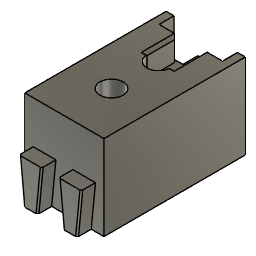
Connector_piece (Autodesk Fusion 360 design; units mm, degrees)
Autodesk Fusion 360 part; units mm, degrees
note: some values were not read from the file. Set by a fixed rule: which sketch regions a step uses.
sketch "Sketch1" plane through (0, 0, 0) normal (0, 1, 0) x (1, 0, 0)
  line L0 (0, 0) -> (28, 0)
  line L1 (28, 0) -> (28, -30)
  line L2 (28, -30) -> (0, -30)
  line L3 (0, -30) -> (0, 0)
  dimension "d1" = 28
  dimension "d2" = 30
  constraint horizontal L0
  constraint vertical L1
  constraint horizontal L2
  constraint vertical L3
  constraint coincident L0.start L3.end
  measures "d1" distance of L0.start L0.end
  measures "d2" distance of L0.start L2.end
extrude "Extrude1" add sketch "Sketch1" along normal blind 50
sketch "Sketch3" plane through (0, 0, 30) normal (0, 0, 1) x (-1, 0, 0)
  line L0 (0, 0) -> (-28, 0)
  line L1 (-28, 0) -> (-28, -50)
  line L2 (-28, -50) -> (0, -50)
  line L3 (0, -50) -> (0, 0)
  line L4 (0, -16.6667) -> (-28, -16.6667)
  line L5 (0, -33.3333) -> (-28, -33.3333)
  circle A0 centre (-14, -33.3333) radius 2
  circle A1 centre (-14, -16.6667) radius 2
  circle A2 centre (-14, -16.6667) radius 4.1
  circle A3 centre (-14, -33.3333) radius 4.1
  dimension "d25" = 16.6667
  dimension "d26" = 16.6667
  dimension "d27" = 4
  dimension "d28" = 4
  dimension "d29" = 8.2
  dimension "d30" = 8.2
  constraint coincident L3 L4.start
  constraint coincident L1 L4.end
  constraint perpendicular L1 L4
  constraint coincident L3 L5.start
  constraint coincident L1 L5.end
  constraint perpendicular L1 L5
  constraint midpoint L5 A0.centre
  constraint midpoint L4 A1.centre
  constraint concentric A1 A2
  constraint concentric A0 A3
  measures "d25" distance of L0 L4
  measures "d26" distance of L2 L5
  measures "d27" diameter of A0
  measures "d28" diameter of A1
  measures "d29" diameter of A2
  measures "d30" diameter of A3
extrude "Extrude5" cut sketch "Sketch3" against normal blind 30 contours L4 A1 | L4 A1 | L5 A0 | L5 A0
sketch "Sketch2" plane through (0, 50, 0) normal (0, 1, 0) x (-1, 0, 0)
  line L0 (0, 30) -> (-28, 30)
  line L1 (-28, 30) -> (-28, 0)
  line L2 (-28, 0) -> (0, 0)
  line L3 (0, 0) -> (0, 30)
  line L4 (-28, 30) -> (-14, 30) construction
  line L5 (-14, 30) -> (-14, 0) construction
  line L6 (-14, 0) -> (-28, 0) construction
  line L7 (-28, 0) -> (-28, 30) construction
  line L8 (-21, 30) -> (-21, 0) construction
  line L9 (-21, 0) -> (-23.5, 0)
  line L10 (-21, 0) -> (-18.5, 0)
  line L11 (-21, 15) -> (-25, 15)
  line L12 (-25, 15) -> (-23.5, 0)
  line L13 (-21, 0) -> (-18.5, 0)
  line L14 (-21, 0) -> (-23.5, 0)
  line L15 (-17, 15) -> (-18.5, 0)
  line L16 (-21, 15) -> (-17, 15)
  line L17 (-11, 15) -> (-9.5, 0)
  line L18 (-7, 15) -> (-11, 15)
  line L19 (-7, 15) -> (-3, 15)
  line L20 (-3, 15) -> (-4.5, 0)
  line L21 (-7, 0) -> (-4.5, 0)
  line L22 (-7, 0) -> (-9.5, 0)
  line L23 (-21, 15.5) -> (-16.4475, 15.5)
  line L24 (-16.4475, 15.5) -> (-18.0475, -0.5)
  line L25 (-21, -0.5) -> (-18.0475, -0.5)
  line L26 (-21, -0.5) -> (-23.9525, -0.5)
  line L27 (-25.5525, 15.5) -> (-23.9525, -0.5)
  line L28 (-21, 15.5) -> (-25.5525, 15.5)
  line L29 (-7, -0.5) -> (-9.9525, -0.5)
  line L30 (-11.5525, 15.5) -> (-9.9525, -0.5)
  line L31 (-7, 15.5) -> (-11.5525, 15.5)
  line L32 (-7, 15.5) -> (-2.4475, 15.5)
  line L33 (-2.4475, 15.5) -> (-4.0475, -0.5)
  line L34 (-7, -0.5) -> (-4.0475, -0.5)
  line L35 (-25.5525, 15.5) -> (-25.5525, 30)
  line L36 (-2.4475, 15.5) -> (-2.4475, 30)
  line L37 (-16.4475, 15.5) -> (-16.4475, 30)
  line L38 (-11.5525, 15.5) -> (-11.5525, 30)
  line L39 (-28, 30) -> (-28, 22)
  line L40 (0, 30) -> (0, 22)
  line L41 (0, 22) -> (-9.2, 22)
  line L42 (-28, 22) -> (-18.8, 22)
  line L43 (-18.8, 22) -> (-18.8, 30)
  line L44 (-9.2, 22) -> (-9.2, 30)
  line L45 (-18.8, 22) -> (-9.2, 22)
  line L46 (-7, 15.2) -> (-11.221, 15.2)
  line L47 (-11.221, 15.2) -> (-9.681, -0.2)
  line L48 (-7, -0.2) -> (-9.681, -0.2)
  line L49 (-7, -0.2) -> (-4.319, -0.2)
  line L50 (-2.779, 15.2) -> (-4.319, -0.2)
  line L51 (-7, 15.2) -> (-2.779, 15.2)
  line L52 (-21, 15.2) -> (-16.779, 15.2)
  line L53 (-16.779, 15.2) -> (-18.319, -0.2)
  line L54 (-21, -0.2) -> (-18.319, -0.2)
  line L55 (-21, -0.2) -> (-23.681, -0.2)
  line L56 (-25.221, 15.2) -> (-23.681, -0.2)
  line L57 (-21, 15.2) -> (-25.221, 15.2)
  line L58 (-25.221, 15.2) -> (-25.221, 30)
  line L59 (-16.779, 15.2) -> (-16.779, 30)
  line L60 (-11.221, 15.2) -> (-11.221, 30)
  line L61 (-2.779, 15.2) -> (-2.779, 30)
  dimension "d5" = 2.5
  dimension "d6" = 2.5
  dimension "d7" = 4
  dimension "d8" = 15
  dimension "d9" = -0.5
  dimension "d16" = 8
  dimension "d17" = 8
  dimension "d18" = 9.2
  dimension "d19" = 9.2
  dimension "d20" = 8
  dimension "d37" = 0.2
  dimension "d38" = 0.2
  dimension "d39" = 180
  constraint horizontal L4
  constraint vertical L5
  constraint horizontal L6
  constraint vertical L7
  constraint midpoint L2 L5.end
  constraint coincident L0.end L1.start
  constraint midpoint L4 L8.start
  constraint midpoint L6 L8.end
  constraint perpendicular L8 L9
  constraint perpendicular L8 L10
  constraint coincident L8 L11.start
  constraint perpendicular L8 L11
  constraint symmetric L9.start L8 L10.start
  constraint symmetric L8 L9.end L10.end
  constraint symmetric L8 L10.end L9.end
  constraint symmetric L8 L11.start L16.start
  constraint symmetric L8 L11.end L15.start
  constraint symmetric L5 L8.end L21.start
  constraint symmetric L5 L9.end L20.end
  constraint symmetric L5 L11.start L18.start
  constraint symmetric L5 L11.end L19.end
  constraint symmetric L5 L10.end L17.end
  constraint symmetric L5 L15.start L17.start
  constraint vertical L35
  constraint coincident L4 L35.end
  constraint symmetric L5 L27.start L32.end
  constraint symmetric L5 L35.end L36.end
  constraint symmetric L8 L27.start L23.end
  constraint symmetric L8 L35.end L37.end
  constraint symmetric L5 L23.end L30.start
  constraint symmetric L5 L37.end L38.end
  constraint perpendicular L4 L39
  constraint coincident L0.start L3.end
  constraint perpendicular L0 L40
  constraint perpendicular L40 L41
  constraint perpendicular L35 L42
  constraint vertical L43
  constraint coincident L0 L44.end
  constraint perpendicular L0 L44
  constraint vertical L58
  constraint coincident L4 L58.end
  constraint coincident L4 L59.end
  constraint symmetric L5 L52.end L46.end
  constraint symmetric L5 L56.start L50.start
  constraint symmetric L5 L58.end L61.end
  constraint symmetric L5 L59.end L60.end
  measures "d5" distance of L8.end L9.end
  measures "d6" distance of L8.end L10.end
  measures "d7" distance of L11.start L11.end
  measures "d8" distance of L9 L11
  measures "d16" distance of L0.end L39.end
  measures "d17" distance of L0.start L40.end
  measures "d18" distance of L40.end L41.end
  measures "d19" distance of L39.end L42.end
  measures "d20" distance of L42.end L43.end
  measures "d39" angle of L58 L59
extrude "Extrude6" cut sketch "Sketch3" against normal blind 24 contours L4 A1 A2 | L4 A1 A2 | L5 A0 A3 | L5 A0 A3
chamfer "Chamfer4" distance 1.8 angle 45 2 edges at (15.8647, 34.0566, 6) (15.8647, 17.3899, 6)
extrude "Extrude4" cut sketch "Sketch2" against normal blind 16 contours L0 L44 L45 L60 | L0 L38 L45 L60 | L0 L37 L38 L45 | L0 L37 L45 L59 | L0 L43 L45 L59
extrude "Extrude3" add sketch "Sketch2" against normal blind 5 from surface at -50 contours L2 L17 L18 L19 L20 L21 L22 | L2 L9 L10 L11 L12 L13 L14 L15 L16
chamfer "Chamfer1" distance 0.5 angle 45 4 edges at (3.75, -5, 7.5) (10.25, -5, 7.5) (17.75, -5, 7.5) (24.25, -5, 7.5)
extrude "Extrude2" cut sketch "Sketch2" against normal blind 5.3 contours L0 L41 L44 L61 | L0 L44 L45 L60 | L31 L32 L41 L45 L60 L61 | L31 L32 L46 L51 L60 L61 | L2 L17 L18 L19 L20 L46 L47 L50 L51 | L2 L17 L18 L19 L20 L21 L22 | L0 L43 L45 L59 | L0 L42 L43 L58 | L23 L28 L42 L45 L58 L59 | L23 L28 L52 L57 L58 L59 | L2 L9 L10 L13 L14 L53 L54 L55 L56 | L2 L11 L12 L15 L16 L52 L53 L56 L57 | L2 L9 L10 L11 L12 L13 L14 L15 L16
chamfer "Chamfer2" distance 1 angle 45 4 edges at (18.8, 39.35, 30) (18.4227, 34, 30) (9.5773, 34, 30) (9.2, 39.35, 30)
chamfer "Chamfer3" distance 1 angle 45 2 edges at (18.8, 44.7, 25.5) (9.2, 44.7, 25.5)
chamfer "Chamfer6" distance 0.7 angle 45 2 edges at (18.0454, 34, 25.5) (9.9546, 34, 25.5)
ref_plane "WorkPlane1" through (14, 25, 15) normal (1, 0, 0) x (0, 0, -1)
equation "d25 = ( 50 / 3 ) * 1 mm"
equation "d26 = ( 50 / 3 ) * 1 mm"
